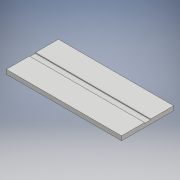
# Autodesk Inventor part: Zijplaat 1
Saved by Autodesk Inventor 2018.3 (Build 223284000, 284)
## iProperties
Created: 2020-11-10
Part Number: Zijplaat 1
Material: Generic
Document SubType Name: Modeling
Designer: daanv
Density: 1 g/cm^3
Appearance: Default
Author: daanv
Autodesk Inventor part; units mm, degrees
ref_plane "YZ Plane" through (0, 0, 0) normal (1, 0, 0) x (0, 1, 0)
ref_plane "XZ Plane" through (0, 0, 0) normal (0, 1, 0) x (-1, 0, 0)
ref_plane "XY Plane" through (0, 0, 0) normal (0, 0, 1) x (1, 0, 0)
sketch "Sketch1" plane through (0, 0, 0) normal (0, 0, 1) x (1, 0, 0)
  line L0 (0, 0) -> (0, 14.7)
  line L1 (0, 14.7) -> (32.5, 14.7)
  line L2 (32.5, 14.7) -> (32.5, 0)
  line L3 (32.5, 0) -> (0, 0)
  dimension "d0" = 14.7
  dimension "d1" = 32.5
  constraints: 8 end point, 3 perpendicular, 1 vertical
  measures "d0" distance of L0.start L0.end
  measures "d1" distance of L0.end L1.end
extrude "Extrusion1" add sketch "Sketch1" along normal blind 1.2
sketch "Sketch2" plane through (0, 0, 1.2) normal (0, 0, 1) x (1, 0, 0)
  line L0 (0, 14.7) -> (0, 0) projected
  line L1 (0, 0) -> (32.5, 0) projected
  line L2 (0, 8.2) -> (32.5, 8.2)
  line L3 (32.5, 8.2) -> (32.5, 6.5)
  line L4 (32.5, 6.5) -> (0, 6.5)
  line L5 (0, 6.5) -> (0, 8.2)
  dimension "d4" = 32.5
  dimension "d5" = 1.7
  dimension "d6" = 6.5
  constraints: 8 end point, 3 parallel, 1 horizontal, 1 perpendicular, 1 point on line
  measures "d4" distance of L3.end L4.end
  measures "d5" distance of L2.end L3.end
  measures "d6" distance of L0.start L2.start
extrude "Extrusion2" cut sketch "Sketch2" against normal blind 0.2
body "Solid1"
